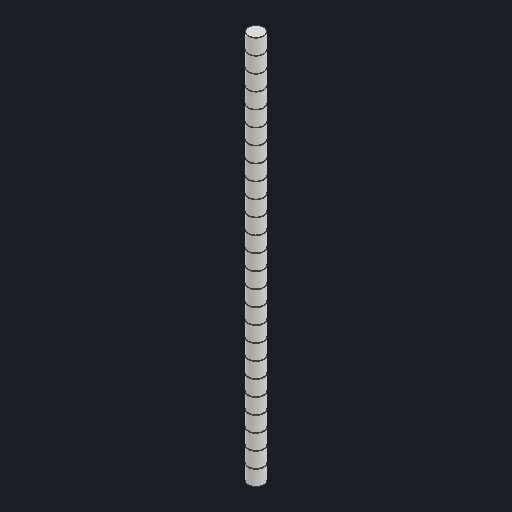
# Autodesk Inventor part: Post
Saved by Autodesk Inventor 2023.1 (Build 271208000, 208)
## iProperties
Created: 2022-12-06
Part Number: Post
Material: Generic
Document SubType Name: Modeling
Designer: aubrey-work
Density: 1 g/cm^3
Appearance: Default
postDiameter: 1.000 in
graduationHeight: 1.000 in
Author: aubrey-work
Autodesk Inventor part; units mm, degrees
ref_plane "YZ Plane" through (0, 0, 0) normal (1, 0, 0) x (0, 1, 0)
ref_plane "XZ Plane" through (0, 0, 0) normal (0, 1, 0) x (-1, 0, 0)
ref_plane "XY Plane" through (0, 0, 0) normal (0, 0, 1) x (1, 0, 0)
sketch "Sketch1" plane through (0, 0, 0) normal (0, 1, 0) x (-1, 0, 0)
  circle A0 centre (0, 0) radius 12.7
  dimension "postDiameter" = 25.4
  constraints: 1 centre point, 1 coincident
  measures "postDiameter" diameter of A0
extrude "Extrude:graduation" add sketch "Sketch1" along normal blind 25.4
chamfer "Chamfer1" distance 0.508 angle 45 2 edges at (12.7, 25.4, 0) (12.7, 0, 0)
pattern_linear "Rectangular Pattern1" count 25 spacing 25.4 along (0, 1, 0)
equation "\"d3\" = 0.02 * postDiameter"
equation "\"d8\" = graduationHeight"
equation "\"graduationHeight\" = 25.4"
